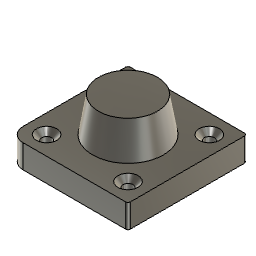
Base_Rear_2x_Front_Left (Autodesk Fusion 360 design; units mm, degrees)
Autodesk Fusion 360 part; units mm, degrees
note: some values were not read from the file. Set by a fixed rule: which sketch regions a step uses.
sketch "Skizze1" plane through (0, 0, 0) normal (0, 0, 1) x (1, 0, 0)
  line L0 (0, 0) -> (50.5, 0)
  line L1 (50.5, 0) -> (50.5, 50.5)
  line L2 (50.5, 50.5) -> (0, 50.5)
  line L3 (0, 50.5) -> (0, 0)
  line L4 (50.5, 0) -> (50.5, 5)
  line L5 (50.5, 5) -> (50.5, 8.5)
  line L6 (50.5, 8.5) -> (50.5, 13.5)
  dimension "d1" = 50.5
  dimension "d2" = 50.5
  constraint horizontal L0
  constraint vertical L1
  constraint horizontal L2
  constraint vertical L3
  constraint coincident L0.start L3.end
  constraint perpendicular L0 L4
  constraint coincident L1 L6.end
  measures "d1" distance of L0.start L0.end
  measures "d2" distance of L0.start L2.end
extrude "Extrusion1" add sketch "Skizze1" along normal blind 10
sketch "Skizze2" plane through (0, 0, 10) normal (0, 0, 1) x (-1, 0, 0)
  line L0 (-50.5, 0) -> (-50.5, -50.5)
  line L1 (-50.5, -50.5) -> (0, -50.5)
  line L2 (0, -50.5) -> (0, 0)
  line L3 (0, 0) -> (-50.5, 0)
  line L4 (0, 0) -> (-25.25, 0)
  line L5 (-25.25, 0) -> (-25.25, -50.5)
  circle A0 centre (-25.25, -25.25) radius 15
  line L6 (0, 0) -> (0, -8)
  line L7 (0, -8) -> (-8, -8)
  line L8 (-50.5, -5) -> (-50.5, 0)
  line L9 (-50.5, 0) -> (-50.5, -8)
  line L10 (-50.5, -8) -> (-42.5, -8)
  line L11 (-50.5, -50.5) -> (-50.5, -42.5)
  line L12 (-50.5, -42.5) -> (-42.5, -42.5)
  line L13 (-5, -50.5) -> (0, -50.5)
  line L14 (0, -50.5) -> (-8, -50.5)
  line L15 (-8, -50.5) -> (-8, -42.5)
  dimension "d18" = 25.25
  dimension "d19" = 30
  dimension "d20" = 8
  dimension "d21" = 8
  dimension "d22" = 8
  dimension "d23" = 8
  dimension "d24" = 8
  dimension "d25" = 8
  dimension "d26" = 8
  dimension "d27" = 8
  constraint coincident L2.end L3.start
  constraint perpendicular L2 L4
  constraint coincident L1 L5.end
  constraint perpendicular L1 L5
  constraint midpoint L5 A0.centre
  constraint perpendicular L4 L6
  constraint perpendicular L6 L7
  constraint coincident L3 L0.start
  constraint perpendicular L3 L8
  constraint perpendicular L9 L10
  constraint coincident L0.end L1.start
  constraint perpendicular L1 L11
  constraint perpendicular L11 L12
  constraint coincident L2 L1.end
  constraint perpendicular L14 L15
  measures "d18" distance of L2.end L4.end
  measures "d19" diameter of A0
  measures "d20" distance of L2.end L6.end
  measures "d21" distance of L6.end L7.end
  measures "d22" distance of L0.start L9.end
  measures "d23" distance of L9.end L10.end
  measures "d24" distance of L0.end L11.end
  measures "d25" distance of L11.end L12.end
  measures "d26" distance of L1.end L14.end
  measures "d27" distance of L14.end L15.end
extrude "Extrusion2" add sketch "Skizze2" along normal blind 14.8 contours L5 A0 | L5 A0
chamfer "Fase1" distance 2.5 distance2 14.8 1 edges at (39.2349, 30.6742, 24.8) measured on face at (22.0767, 28.4139, 24.8)
hole "Bohrung1" at (8, 8, 10) at (42.5, 8, 10) at (42.5, 42.5, 10) at (8, 42.5, 10) direction (0, 0, -1) diameter 4.2 depth 13 tip angle 180 countersink diameter 8.6 countersink angle 90
fillet "Abrundung1" radius 6 1 edges at (0, 0, 5)
fillet "Fillet3" radius 1 3 edges at (50.5, 0, 5) (50.5, 50.5, 5) (0, 50.5, 5)
